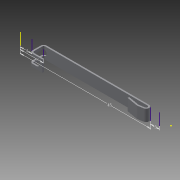
# Autodesk Inventor part: snip
Saved by Autodesk Inventor 2015 (Build 190159000, 159)
## iProperties
Created: 2014-12-01
Part Number: snip
Material: 常规
Document SubType Name: 钣金
Designer: zenkr
Density: 1 g/cm^3
Sheet Metal Rule: 默认_mm
Appearance: 默认
Author: zenkr
Autodesk Inventor part; units mm, degrees
ref_plane "YZ Plane" through (0, 0, 0) normal (1, 0, 0) x (0, 1, 0)
ref_plane "XZ Plane" through (0, 0, 0) normal (0, 1, 0) x (-1, 0, 0)
ref_plane "XY Plane" through (0, 0, 0) normal (0, 0, 1) x (1, 0, 0)
sketch "草图1" plane through (0, 0, 0) normal (0, 1, 0) x (-1, 0, 0)
  line L0 (0, 0) -> (0, -2)
  line L1 (0, 0) -> (0, 2)
  line L2 (0, 2) -> (52, 2)
  line L3 (52, 2) -> (52, -2)
  line L4 (52, -2) -> (0, -2)
  line L5 (43.9181, 0) -> (50, 0) construction
  line L6 (43.9181, -1) -> (50, -1)
  line L7 (50, 1) -> (43.9181, 1)
  arc A0 (43.9181, 1) -> (43.9181, -1) centre (43.9181, 0) ccw
  arc A1 (50, -1) -> (50, 1) centre (50, 0) ccw
  point P0 (46.9591, 0)
  dimension "d0" = 2
  dimension "d1" = 2
  dimension "d2" = 52
  dimension "d39" = 2
  measures "d0" distance of L0.start L0.end
  measures "d1" distance of L0.start L1.end
  measures "d2" distance of L1.end L2.end
  measures "d39" distance from line of L3 L5.end
extrude "平板1" add sketch "草图1" along normal blind 0.5
sketch "草图2" plane through (0, 0, 0) normal (0, 1, 0) x (-1, 0, 0)
  line L0 (48, -2) -> (48, 2)
  line L1 (52, -2) -> (52, 2) projected
  line L2 (44, -2) -> (44, 2)
  line L3 (7, -2) -> (7, 2)
  line L4 (4, -2) -> (4, 2)
  point P0 (0, 0)
  dimension "d4" = 4
  dimension "d5" = 8
  dimension "d6" = 45
  dimension "d7" = 3
  constraints: 8 end point, 4 vertical
  measures "d4" distance between parallel lines of L0 L1
  measures "d5" distance between parallel lines of L2 L1
  measures "d6" distance between parallel lines of L3 L1
  measures "d7" distance between parallel lines of L4 L3
fold "折叠1" angle 90 bend radius 0.5 thickness 0.5 k factor 0.44 line from (-48, 0, -2) to (-48, 0, 2) line at bend centre moving side (-1, 0, 0) folds toward (0, -1, 0)
fold "折叠2" angle 90 bend radius 0.5 thickness 0.5 k factor 0.44 line from (-44, 0, -2) to (-44, 0, 2) line at bend centre moving side (-1, 0, 0) folds toward (0, -1, 0)
fold "折叠4" angle 20 bend radius 0.5 thickness 0.5 k factor 0.44 line from (-4, 0, -2) to (-4, 0, 2) line at bend centre moving side (1, 0, 0) folds toward (0, -1, 0)
fold "折叠5" angle 170 bend radius 0.5 thickness 0.5 k factor 0.44 line from (-7, 0, -2) to (-7, 0, 2) line at bend centre moving side (1, 0, 0) folds toward (0, -1, 0)
equation "\"d8\" = 折弯释压宽度"
equation "\"d9\" = 折弯释压深度"
equation "\"d10\" = 最小余量"
equation "\"d11\" = 折弯半径"
equation "\"d13\" = 折弯半径"
equation "\"d14\" = 折弯释压宽度"
equation "\"d15\" = 折弯释压深度"
equation "\"d16\" = 最小余量"
equation "\"d17\" = 折弯半径"
equation "\"d19\" = 折弯半径"
equation "\"d27\" = 折弯释压宽度"
equation "\"d28\" = 折弯释压深度"
equation "\"d29\" = 最小余量"
equation "\"d30\" = 折弯半径"
equation "\"d32\" = 折弯半径"
equation "\"d33\" = 折弯释压宽度"
equation "\"d34\" = 折弯释压深度"
equation "\"d35\" = 最小余量"
equation "\"d36\" = 折弯半径"
equation "\"d38\" = 折弯半径"
equation "\"折弯半径\" = 厚度"
equation "\"折弯释压宽度\" = 厚度"
equation "\"折弯释压深度\" = 0.5 * 厚度"
equation "\"拐角释压尺寸\" = 4 * 厚度"
equation "\"最小余量\" = 2 * 厚度"
equation "\"过渡半径\" = 折弯半径"
equation "\"Jacobi半径尺寸\" = 折弯半径"
equation "\"间隙大小\" = 厚度"
equation "\"d3\" = 折弯半径"
equation "\"厚度\" = 0.5"
